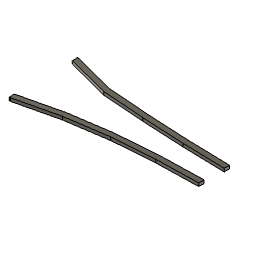
ArmSideView v2 (Autodesk Fusion 360 design; units mm, degrees)
Autodesk Fusion 360 part; units mm, degrees
sketch "Sketch1" plane through (0, 0, 0) normal (0, 0, 1) x (1, 0, 0)
  line L0 (16.6494, -187.3513) -> (56.6494, -197.7413)
  line L1 (56.6494, -197.7413) -> (96.6494, -200.7413)
  line L2 (96.6494, -200.7413) -> (136.6494, -202.7413)
  line L3 (136.6494, -202.7413) -> (176.6494, -203.7413)
  line L4 (16.6494, -242.1313) -> (56.6494, -232.7413)
  line L5 (56.6494, -232.7413) -> (96.6494, -226.7413)
  line L6 (96.6494, -226.7413) -> (136.6494, -223.7413)
  line L7 (136.6494, -223.7413) -> (176.6494, -222.7413)
  line L8 (17.9064, -182.5119) -> (57.4715, -192.7889)
  line L9 (57.4715, -192.7889) -> (96.9613, -195.7506)
  line L10 (96.9613, -195.7506) -> (136.8367, -197.7444)
  line L11 (17.7921, -246.999) -> (57.5932, -237.6557)
  line L12 (57.5932, -237.6557) -> (97.208, -231.7134)
  line L13 (97.208, -231.7134) -> (136.899, -228.7366)
  line L14 (16.6494, -187.3513) -> (16.6494, -182.3513)
  line L15 (16.6494, -242.1313) -> (16.6494, -247.1313)
  line L16 (176.6494, -203.7413) -> (176.6494, -198.7413)
  line L17 (176.6494, -222.7413) -> (176.6494, -227.7413)
  line L18 (17.9064, -182.5119) -> (16.6494, -182.3513)
  line L19 (17.7921, -246.999) -> (16.6494, -247.1313)
  line L20 (176.6494, -227.7413) -> (136.899, -228.7366)
  line L21 (176.6494, -198.7413) -> (136.8367, -197.7444)
  dimension "d5" = 54.78
  dimension "d17" = 5
  dimension "d18" = 5
  dimension "d19" = 5
  dimension "d20" = 5
  constraint vertical L14
  constraint vertical L15
  constraint vertical L17
  measures "d5" distance of L0.start L4.start
  measures "d17" distance of L0.start L14.end
  measures "d18" distance of L4.start L15.end
  measures "d19" distance of L7.end L17.end
  measures "d20" distance of L3.end L16.end
extrude "Extrude1" add sketch "Sketch1" along normal blind 3 makes body 1 at (43.6306, -237.5094, 0) makes body 2 at (43.5901, -192.6272, 0)
